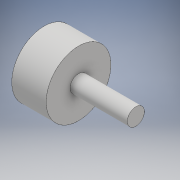
# Autodesk Inventor part: 模擬配重
Saved by Autodesk Inventor 2017 (Build 210142000, 142)
## iProperties
Part Number: 模擬配重
Material: 一般
Document SubType Name: Modeling
Designer: Brian
Mass: 130 g
Surface Area: 230.407 cm^2
Volume: 205.745 cm^3
Density: 0.631851 g/cm^3
Appearance: 預設
Author: Brian
Autodesk Inventor part; units mm, degrees
ref_plane "YZ Plane" through (0, 0, 0) normal (1, 0, 0) x (0, 1, 0)
ref_plane "XZ Plane" through (0, 0, 0) normal (0, 1, 0) x (-1, 0, 0)
ref_plane "XY Plane" through (0, 0, 0) normal (0, 0, 1) x (1, 0, 0)
sketch "草圖1" plane through (0, 0, 0) normal (0, 1, 0) x (-1, 0, 0)
  line L0 (0, 0) -> (108, 0)
  line L1 (108, 0) -> (108, -10)
  line L2 (108, -10) -> (0, -10)
  line L3 (0, -10) -> (0, 0)
  line L4 (108, -10) -> (67.4678, -10)
  line L5 (67.4678, -10) -> (67.4678, -38.0698)
  line L6 (67.4678, -38.0698) -> (108, -38.0698)
  line L7 (108, -38.0698) -> (108, -10)
  dimension "d0" = 108
  dimension "d2" = 10
  constraints: 16 end point, 4 parallel, 2 horizontal, 2 perpendicular
  measures "d0" distance of L0.start L0.end
  measures "d2" distance of L0.end L1.end
revolve "迴轉1" add sketch "草圖1" angle 360 about axis through (0, 0, 0) along (-1, 0, 0)
